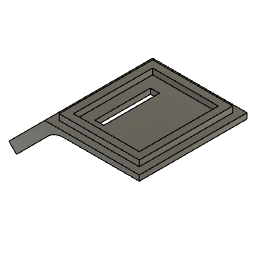
weather_station_light_sensor_base v16 (Autodesk Fusion 360 design; units mm, degrees)
Autodesk Fusion 360 part; units mm, degrees
sketch "Sketch1" plane through (0, 0, 0) normal (0, 0, 1) x (1, 0, 0)
  line L0 (0, 0) -> (26.3, 0)
  line L1 (26.3, 0) -> (26.3, 30)
  line L2 (26.3, 30) -> (0, 30)
  line L3 (0, 30) -> (0, 0)
  line L4 (2, 28) -> (24.3, 28)
  line L5 (24.3, 28) -> (24.3, 2)
  line L6 (24.3, 2) -> (2, 2)
  line L7 (2, 2) -> (2, 28)
  line L8 (4, 26) -> (22.3, 26)
  line L9 (22.3, 26) -> (22.3, 4)
  line L10 (22.3, 4) -> (4, 4)
  line L11 (4, 4) -> (4, 26)
  dimension "d1" = 26.3
  dimension "d2" = 30
  dimension "d3" = 2
  dimension "d4" = 2
  dimension "d5" = 2
  dimension "d6" = 2
  dimension "d7" = 2
  dimension "d8" = 2
  dimension "d9" = 2
  dimension "d10" = 2
  dimension "d45" = 17.3
  constraint horizontal L0
  constraint vertical L1
  constraint horizontal L2
  constraint vertical L3
  constraint coincident L0.start L3.end
  constraint horizontal L4
  constraint vertical L5
  constraint horizontal L6
  constraint vertical L7
  constraint horizontal L8
  constraint vertical L9
  constraint horizontal L10
  constraint vertical L11
  measures "d1" distance of L0.start L0.end
  measures "d2" distance of L0.start L2.end
  measures "d3" distance of L1 L5
  measures "d4" distance of L2 L4
  measures "d5" distance of L3 L7
  measures "d7" distance of L5 L9
  measures "d8" distance of L4 L8
  measures "d9" distance of L7 L11
  measures "d16" distance of L0.end
extrude "Extrude2" add sketch "Sketch1" along normal blind 1.5 makes body 1 at (10.1, 18.6667, 0) makes body 2 at (25.6333, 10.6667, 0)
extrude "Extrude1" add sketch "Sketch1" along normal blind 3.12 contours L4 L5 L6 L7 bodies 1 2
sketch "Sketch2" plane through (0, 0, 1.5) normal (0, 0, 1) x (-1, 0, 0)
  line L0 (-6.9, -22.5) -> (-9.4, -22.5)
  line L1 (-9.4, -22.5) -> (-9.4, -7)
  line L2 (-9.4, -7) -> (-6.9, -7)
  line L3 (-6.9, -7) -> (-6.9, -22.5)
  line L4 (-4, -4) -> (-22.3, -4)
  line L5 (-22.3, -4) -> (-22.3, -26)
  line L6 (-22.3, -26) -> (-4, -26)
  line L7 (-4, -26) -> (-4, -4)
  line L8 (-24.3, -2) -> (-2, -2)
  line L9 (-2, -2) -> (-2, -28)
  line L10 (-2, -28) -> (-24.3, -28)
  line L11 (-24.3, -28) -> (-24.3, -2)
  line L12 (0, -30) -> (0, 0)
  line L13 (0, 0) -> (-26.3, 0)
  line L14 (-26.3, 0) -> (-26.3, -30)
  line L15 (-26.3, -30) -> (0, -30)
  line L16 (-4.4, -23) -> (-4.4, -7)
  dimension "d15" = 15.5
  dimension "d16" = 2.5
  dimension "d39" = 2.9
  dimension "d40" = 6.9
  dimension "d41" = 4.9
  dimension "d43" = 4.4
  dimension "d44" = 2.5
  constraint horizontal L0
  constraint vertical L1
  constraint horizontal L2
  constraint vertical L3
  constraint vertical L16
  measures "d15" distance of L0.start L2.end
  measures "d16" distance of L0.start L0.end
  measures "d39" distance of L3 L7
  measures "d40" distance of L3 L12
  measures "d41" distance of L3 L9
  measures "d43" distance of L12 L16
  measures "d44" distance of L3 L16
extrude "Extrude3" cut sketch "Sketch2" against normal blind 3 contours L0 L1 L2 L3 bodies 1
sketch "Sketch3" plane through (0, 0, 0) normal (0, -1, 0) x (1, 0, 0)
  line L0 (0, 0) -> (26.3, 0)
  line L1 (26.3, 0) -> (26.3, 1.5)
  line L2 (26.3, 1.5) -> (0, 1.5)
  line L3 (0, 1.5) -> (0, 0)
  line L4 (0, 1.5) -> (-9.9853, -8.4853)
  line L5 (-9.9853, -8.4853) -> (-7.864, -10.6066)
  line L6 (-7.864, -10.6066) -> (2.7426, 0)
  dimension "d21" = 3
  dimension "d32" = 15
  dimension "d35" = 135
  constraint coincident L2.end L3.start
  constraint perpendicular L4 L5
  constraint coincident L0 L6.end
  constraint perpendicular L5 L6
  measures "d21" distance of L4.end L5.end
  measures "d32" distance of L5.end L6.end
  measures "d35" angle of L0 L6
extrude "Extrude4" add sketch "Sketch3" against normal blind 30 contours L0 L3 L4 L5 L6 bodies 1
sketch "Sketch4" plane through (-0.75, 0, 0.75) normal (-0.707107, 0, 0.707107) x (0, -1, 0)
  line L0 (0, -13.0607) -> (0, 1.0607)
  line L1 (0, 1.0607) -> (-30, 1.0607)
  line L2 (-30, 1.0607) -> (-30, -13.0607)
  line L3 (-30, -13.0607) -> (0, -13.0607)
  circle A0 centre (-20, -7.9903) radius 1.6
  circle A1 centre (-10, -7.9903) radius 1.6
  dimension "d24" = 3.2
  dimension "d25" = 3.2
  dimension "d26" = 10
  dimension "d27" = 10
  dimension "d29" = 9.051
  measures "d24" diameter of A0
  measures "d25" diameter of A1
  measures "d26" distance of A0.centre A1.centre
  measures "d27" distance of L0 A1.centre
  measures "d29" distance of L1 A0.centre
extrude "Extrude5" cut sketch "Sketch4" against normal blind 5 contours A0 | A1 bodies 1
fillet "Fillet2" radius 6 1 edges at (2.7426, 15, 0) on bodies 1
component "Component" placed x (1, 0, 0) y (0, 1, 0) z (0, 0, 1) at (0, 0, 0)
equation "d4 = d3"
equation "d5 = d3"
equation "d6 = d3"
equation "d8 = d7"
equation "d9 = d7"
equation "d10 = d7"
equation "d11 = 1.5 mm + 1.62 mm"
equation "d25 = d24"
equation "d27 = ( 30 mm - d26 ) / 2"
equation "d29 = ( 6.4 / sin(45 °) ) * 1 mm"
equation "d35 = 135 °"
